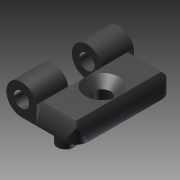
# Autodesk Inventor part: HHPSJC5-r
Saved by Autodesk Inventor 2011 SP1 (Build 150282100, 282)
## iProperties
Created: 2015-01-26
Part Number: HHPSJC5-r
Catalog Web Link: www.cadenas.de
Description: HHPSJC-R-Aluminum Detachable Hinges
Vendor: MISUMI
Document SubType Name: Modeling
Designer: PARTuser1
Manufacturer: MISUMI
Mass: 3.57297 g
Surface Area: 24.7715 cm^2
Volume: 3.57297 cm^3
Density: 1 g/cm^3
Category: PARTsolutions
Company: MISUMI
Title: HHPSJC5-r
Author: Cadenas PARTsolutions
Comments: Aluminum Detachable Hinges
PSOL_IDENT_0: {\\10.0.0.236\data_v8\23d-libs\misumi\metric\39_accessories_for_al_extrusions\hhpsjc_r.prj},162 {VTY
PSOL_IDENT_1: P=3D},{NB=HHPSJC5-r},{LINA=HHPSJC5-r},{NN=HHPSJC-R},{DATE=17.11.2014 05:31:05},{GEOMDATE=08.05.2009
PSOL_IDENT_2: 06:06:00},{VERSION=},{LINEID=10},{LINESUBID=-1},{WBVAR=}  {NB=HHPSJC5-r},{LINA=HHPSJC5-r},{KT=DUMMY}
PSOL_IDENT_3: ,{PN=HHPSJC5},{TYPE=HHPSJC},{MATL=Nylon 6},{MATS=304 Stainless Steel},{NO=5},{ALKG=10},{ALN=98},{MAS
PSOL_IDENT_4: S=12.5},{L=32},{W=36},{K=4},{P=24},{J=7.5},{S=21},{ND=5.5},{NC=11},{T=6},{TT=4},{E=10},{R=5.0},{A=5.
PSOL_IDENT_5: 5},{ND1=2.0}
SUPPLIER: MISUMI
ARTICLENO: HHPSJC5-r
BOMINFO: HHPSJC5-r
CREATOR: CADENAS GmbH
Autodesk Inventor part; units mm, degrees
ref_plane "YZ Plane" through (0, 0, 0) normal (1, 0, 0) x (0, 1, 0)
ref_plane "XZ Plane" through (0, 0, 0) normal (0, 1, 0) x (-1, 0, 0)
ref_plane "XY Plane" through (0, 0, 0) normal (0, 0, 1) x (1, 0, 0)
sketch "Sketch_1" plane through (0, 0, 0) normal (0, 0, 1) x (1, 0, 0)
  line L0 (0, -16) -> (0, 16)
  line L1 (0, 16) -> (5, 16)
  line L2 (5, 16) -> (5, -16)
  line L3 (5, -16) -> (0, -16)
  line L4 (0, -16) -> (0, 16)
  constraints: 10 end point
revolve "Revolution1" add sketch "Sketch_1" angle 360 about axis through (0, -16, 0) along (0, -1, 0)
sketch "Sketch_2" plane through (0, 0, 0) normal (0, 1, 0) x (-1, 0, 0)
  line L0 (0, 1) -> (-16, 1)
  arc A0 (-16, 1) -> (-18, -5) centre (-8, -5) ccw
  line L1 (-18, -5) -> (0, -5)
  line L2 (0, -5) -> (0, 1)
  constraints: 6 end point, 2 point on circle, 1 centre point
extrude "Extrusion1" add sketch "Sketch_2" along normal mid plane 32
sketch "Sketch_4" plane through (18, 0, 0) normal (1, 0, 0) x (0, 0, -1)
  line L0 (-5, -32) -> (10, -32)
  line L1 (10, -32) -> (10, 32)
  line L2 (10, 32) -> (-5, 32)
  line L3 (-5, 32) -> (-5, -32)
  line L4 (-1, 14) -> (-1, -14)
  arc A0 (-1, -14) -> (5, -16) centre (5, -6) ccw
  line L5 (5, -16) -> (5, 16)
  arc A1 (5, 16) -> (-1, 14) centre (5, 6) ccw
  constraints: 12 end point, 4 point on circle, 2 centre point
extrude "Extrusion2" cut sketch "Sketch_4" against normal blind 13
sketch "Sketch_6" plane through (0, 0, -5) normal (0, 0, 1) x (1, 0, 0)
  circle A0 centre (10.5, 12) radius 2.75
  constraints: 1 centre point
extrude "Extrusion3" add sketch "Sketch_6" against normal blind 4
sketch "Sketch_5" plane through (0, 0, -5) normal (0, 0, 1) x (1, 0, 0)
  circle A0 centre (10.5, -12) radius 2.75
  constraints: 1 centre point
extrude "Extrusion4" add sketch "Sketch_5" against normal blind 4
sketch "Sketch_7" plane through (10.5, 0, 0) normal (1, 0, 0) x (0, 0, -1)
  line L0 (5, 0) -> (-1, 0)
  line L1 (-1, 0) -> (-1, 5.5)
  line L2 (-1, 5.5) -> (1.75, 2.75)
  line L3 (1.75, 2.75) -> (5, 2.75)
  line L4 (5, 2.75) -> (5, 0)
  line L5 (5, 0) -> (-1, 0)
  constraints: 12 end point
revolve "Revolution2" cut sketch "Sketch_7" angle 360 about axis through (10.5, 0, -5) along (0, 0, -1)
sketch "Sketch_8" plane through (0, 0, 0) normal (0, 0, 1) x (1, 0, 0)
  line L0 (0, -16) -> (0, 16)
  line L1 (0, 16) -> (2.5, 16)
  line L2 (2.5, 16) -> (2.5, -16)
  line L3 (2.5, -16) -> (0, -16)
  line L4 (0, -16) -> (0, 16)
  constraints: 10 end point
revolve "Revolution3" cut sketch "Sketch_8" angle 360 about axis through (0, -16, 0) along (0, -1, 0)
sketch "Sketch_3" plane through (0, 0, 0) normal (0, 0, 1) x (1, 0, 0)
  line L0 (-36, -36) -> (36, -36)
  line L1 (36, -36) -> (36, 36)
  line L2 (36, 36) -> (-36, 36)
  line L3 (-36, 36) -> (-36, -36)
  line L4 (-5, -16) -> (14, -16)
  arc A0 (14, -16) -> (18, -12) centre (14, -12) ccw
  line L5 (18, -12) -> (18, 12)
  arc A1 (18, 12) -> (14, 16) centre (14, 12) ccw
  line L6 (14, 16) -> (-5, 16)
  line L7 (-5, 16) -> (-5, 5.5333)
  line L8 (-5, 5.5333) -> (5, 5.5333)
  line L9 (5, 5.5333) -> (5, -5.5333)
  line L10 (5, -5.5333) -> (-5, -5.5333)
  line L11 (-5, -5.5333) -> (-5, -16)
  constraints: 24 end point, 4 point on circle, 2 centre point
extrude "Extrusion5" cut sketch "Sketch_3" along normal mid plane 10
ref_plane "hhpsjc_r_XY" through (0, 0, 0) normal (0, 1, 0) x (1, 0, 0)
ref_plane "hhpsjc_r_YZ" through (0, 0, 0) normal (1, 0, 0) x (0, 0, -1)
ref_plane "hhpsjc_r_ZX" through (0, 0, 0) normal (0, 0, -1) x (0, 1, 0)
ref_plane "hole2_to_bolt_XY" through (10.5, 0, 1) normal (0, 0, 1) x (1, 0, 0)
ref_plane "hole2_to_bolt_YZ" through (10.5, 0, 1) normal (1, 0, 0) x (0, 1, 0)
ref_plane "hole2_to_bolt_ZX" through (10.5, 0, 1) normal (0, 1, 0) x (0, 0, 1)
ref_plane "nut2_to_bolt_XY" through (10.5, 0, -7) normal (0, 0, 1) x (1, 0, 0)
ref_plane "nut2_to_bolt_YZ" through (10.5, 0, -7) normal (1, 0, 0) x (0, 1, 0)
ref_plane "nut2_to_bolt_ZX" through (10.5, 0, -7) normal (0, 1, 0) x (0, 0, 1)
body "Solid1"
